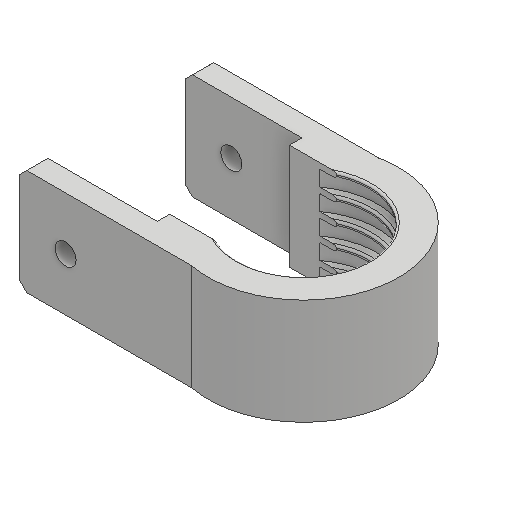
# Autodesk Inventor part: 3DP_ABS_Cable_Pipe_Mount
Saved by Autodesk Inventor 2026.1 (Build 301233000, 233)
## iProperties
Created: 2017-05-29
Part Number: 3DP_ABS_Cable_Pipe_Mount
Material: Ogólny
Document SubType Name: Modeling
Designer: Andrzej
Density: 1 g/cm^3
Appearance: Domyślna
Mass: 4.58563 g
Surface Area: 39.5198 cm^2
Volume: 4.58563 cm^3
Author: Andrzej
Autodesk Inventor part; units mm, degrees
ref_plane "YZ Plane" through (0, 0, 0) normal (1, 0, 0) x (0, 1, 0)
ref_plane "XZ Plane" through (0, 0, 0) normal (0, 1, 0) x (-1, 0, 0)
sketch "Szkic1" plane through (0, 0, 0) normal (0, 0, 1) x (1, 0, 0)
  circle A0 centre (0, 0) radius 10.5
  circle A1 centre (0, 0) radius 13.5
  line L0 (-2.586, 13.25) -> (-27, 13.25)
  line L1 (-27, 13.25) -> (-27, 10.25)
  line L2 (-27, 10.25) -> (-8.7856, 10.25)
  line L3 (-2.586, -13.25) -> (-27, -13.25)
  line L4 (-27, -13.25) -> (-27, -10.25)
  line L5 (-27, -10.25) -> (-8.7856, -10.25)
  line L6 (-10.5, -8.4853) -> (-10.5, -10.25)
  line L7 (-10.5, 8.4853) -> (-10.5, 10.25)
  line L8 (-10.5, 8.4853) -> (-6.1847, 8.4853)
  line L9 (-10.5, -8.4853) -> (-6.1847, -8.4853)
  dimension "d0" = 21
  dimension "d1" = 3
  dimension "d3" = 3
  dimension "d5" = 3
  dimension "d6" = 20.5
  dimension "d8" = 0.25
  dimension "d31" = 16.5
  dimension "d32" = 16.5
  constraints: 20 end point, 8 point on circle, 7 perpendicular, 3 point on line, 2 centre point, 1 coincident, 1 horizontal, 1 parallel, 1 tangent
  measures "d0" diameter of A0
  measures "d1" radial gap between concentric circles of A0 A1
  measures "d3" distance of L0.end L1.end
  measures "d5" distance of L3.end L4.end
  measures "d6" distance between parallel lines of L5 L2
  measures "d8" distance edge to line of A1 L0
  measures "d31" distance between parallel lines of L4 L6
  measures "d32" distance between parallel lines of L7 L1
extrude "Wyciągnięcie proste2" add sketch "Szkic1" along normal blind 15 contours A0 L8 A1 L9 | L7 L2 A1 | A1 L5 L6 | L2 L1 L0 A1 | A1 L3 L4 L5 picked at (12.3911, -0.984)
ref_plane "Płaszczyzna konstrukcyjna1" through (-27, 0, 0) normal (0, -1, 0) x (1, 0, 0)
sketch "Szkic2" plane through (-27, 0, 0) normal (0, -1, 0) x (1, 0, 0)
  line L0 (24.414, 0) -> (24.414, 15) projected
  line L1 (24.414, 15) -> (24.414, 15) projected
  line L2 (24.414, 0) -> (24.414, 15) projected
  line L3 (24.414, 0) -> (24.414, 0) projected
  line L4 (37.5, 15) -> (37.5, 0) projected
  line L5 (20.8153, 15) -> (37.5, 15) projected
  line L6 (37.5, 15) -> (36.6, 15)
  line L7 (36.3, 14.7) -> (36.3, 14.5)
  line L8 (36.6, 14.2) -> (37.5, 14.2)
  arc A0 (36.6, 15) -> (36.3, 14.7) centre (36.6, 14.7) ccw
  arc A1 (36.3, 14.5) -> (36.6, 14.2) centre (36.6, 14.5) ccw
  line L9 (27, 18.0746) -> (27, -3.0124) projected
  point P0 (27, 0)
  point P1 (36.3, 15)
  point P2 (36.3, 14.2)
  dimension "d14" = 1.2
  dimension "d15" = 0.8
  dimension "d16" = 0.3
  constraints: 6 end point, 6 point on line, 4 point on circle, 4 tangent, 2 centre point, 2 perpendicular, 1 equal radius
  measures "d14" distance of L4.start point (36.3, 15)
  measures "d15" distance of point (36.3, 15) point (36.3, 14.2)
  measures "d16" radius of A0
revolve "Obrót1" add sketch "Szkic2" angle 360 about axis through (0, 0, 15) along (0, 0, -1)
pattern_linear "Szyk prostokątny1" count 5 spacing 3 along (0, 0, -1) of "Obrót1"
sketch "Szkic3" plane through (-10.5, 8.4853, 0) normal (-1, 0, 0) x (0, 0, 1)
  line L0 (0, 1.7647) -> (0, 0) projected
  line L1 (0, 0) -> (15, 0) projected
  line L2 (15, 1.7647) -> (15, 0) projected
  line L3 (0, 1.7647) -> (15, 1.7647) projected
  line L4 (0, -16.9706) -> (0, -18.7353) projected
  line L5 (0, -18.7353) -> (15, -18.7353) projected
  line L6 (15, -16.9706) -> (15, -18.7353) projected
  line L7 (0, -16.9706) -> (15, -16.9706) projected
  line L8 (15, 1.7647) -> (15, 0) projected
  line L9 (15, 0) -> (15, -16.9706)
  line L10 (15, 2.0147) -> (15, -16.9706) projected
  line L11 (0, 0) -> (0, -16.9706)
  point P0 (0, -8.4853)
  point P1 (15, -8.4853)
  constraints: 4 end point, 1 collinear, 1 parallel
extrude "Wyciągnięcie proste3" cut sketch "Szkic3" against normal blind 10 contours L1 L9 L7 L11
chamfer "Faza1" distance 1 angle 45 4 edges at (-27, 11.75, 0) (-27, 11.75, 15) (-27, -11.75, 15) (-27, -11.75, 0)
sketch "Szkic4" plane through (-2.586, -13.25, 0) normal (0, -1, 0) x (1, 0, 0)
  line L0 (-23.414, 0) -> (-24.414, 1) projected
  line L1 (-23.414, 0) -> (0, 0) projected
  line L2 (0, 0) -> (0, 15) projected
  line L3 (-23.414, 15) -> (0, 15) projected
  line L4 (-24.414, 14) -> (-23.414, 15) projected
  line L5 (-24.414, 1) -> (-24.414, 14) projected
  point P0 (2.586, 0)
  point P1 (-17.914, 7.5)
  dimension "d36" = 6.5
  dimension "d37" = 7.5
  dimension "d38" = 15
  measures "d36" distance from line of L5 point (-17.914, 7.5)
  measures "d37" distance from line of L3 point (-17.914, 7.5)
  measures "d38" distance between parallel lines of L1 L3
hole "Otwór1" at (-20.5, -13.25, 7.5) direction (0, 1, 0) diameter 3 end through all
equation "\"d32\" = d31"
equation "\"d37\" = 0.5 * d38"
